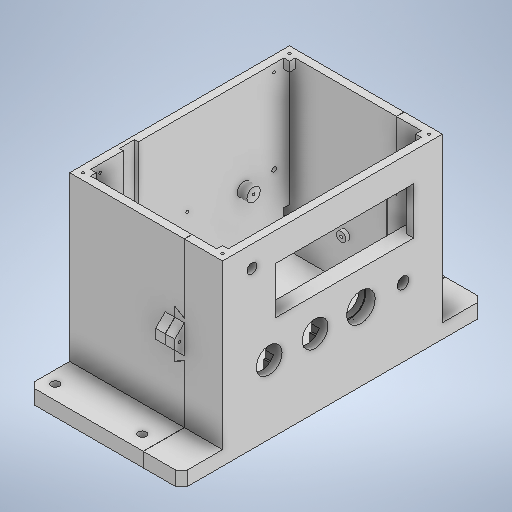
# Autodesk Inventor part: Honigschleuder_Steuerung
Saved by Autodesk Inventor 2025 (Build 290162010, 162A)
## iProperties
Created: 2025-12-04
Part Number: Honigschleuder_Steuerung
Material: Generisch
Document SubType Name: Modeling
Designer: max-h
Density: 1 g/cm^3
Appearance: Vorgabe
Author: max-h
Autodesk Inventor part; units mm, degrees
ref_plane "YZ Plane" through (0, 0, 0) normal (1, 0, 0) x (0, 1, 0)
ref_plane "XZ Plane" through (0, 0, 0) normal (0, 1, 0) x (-1, 0, 0)
ref_plane "XY Plane" through (0, 0, 0) normal (0, 0, 1) x (1, 0, 0)
sketch "Skizze1" plane through (0, 0, 0) normal (0, 1, 0) x (-1, 0, 0)
  line L0 (43.7441, 63.282) -> (-36.2559, 63.282)
  line L1 (-36.2559, 63.282) -> (-36.2559, -51.718)
  line L2 (-36.2559, -51.718) -> (43.7441, -51.718)
  line L3 (43.7441, -51.718) -> (43.7441, 63.282)
  point P0 (0, 0)
  dimension "d0" = 115
  dimension "d1" = 80
  constraints: 8 end point, 2 parallel, 1 horizontal, 1 perpendicular
  measures "d0" distance of L0.end L1.end
  measures "d1" distance of L1.end L2.end
extrude "Extrusion1" add sketch "Skizze1" along normal blind 93
shell "Wandung1" thickness 4 removed faces 1 at (9.5893, 93, -13.3847)
sketch "Skizze2" plane through (36.2559, 0, 63.282) normal (1, 0, 0) x (0, 0, -1)
  line L0 (27.85, 78) -> (100, 78)
  line L1 (100, 78) -> (100, 53.4)
  line L2 (100, 53.4) -> (27.85, 53.4)
  line L3 (27.85, 53.4) -> (27.85, 78)
  line L4 (115, 0) -> (115, 93) projected
  line L5 (0, 0) -> (115, 0) projected
  circle A0 centre (94.375, 35.9) radius 3
  circle A1 centre (72.375, 35.9) radius 7
  circle A2 centre (48.375, 35.9) radius 6.75
  circle A3 centre (24.375, 35.9) radius 6.75
  line L6 (27.85, 78) -> (17.85, 78) construction
  line L7 (17.85, 78) -> (17.85, 43) construction
  line L8 (17.85, 43) -> (27.85, 43) construction
  line L9 (27.85, 43) -> (27.85, 78) construction
  line L10 (94.375, 35.9) -> (24.375, 35.9) construction
  line L11 (0, 93) -> (115, 93) projected
  line L12 (0, 0) -> (0, 93) projected
  line L13 (17.625, 40.8928) -> (17.625, 21.6445) construction
  line L14 (97.375, 42.4272) -> (97.375, 31.7493) construction
  line L15 (94.375, 35.9) -> (97.375, 35.9) construction
  line L16 (24.375, 35.9) -> (17.625, 35.9) construction
  line L17 (57.5, 46.1925) -> (57.5, 22.2697) construction
  line L18 (0, 44.5) -> (0, 23.5685) construction
  line L19 (115, 44.5) -> (115, 22.2697) construction
  circle A4 centre (15.35, 82) radius 2.55
  point P0 (63.282, 0)
  dimension "d11" = 6
  dimension "d5" = 72.15
  dimension "d6" = 24.6
  dimension "d7" = 15
  dimension "d12" = 14
  dimension "d13" = 13.5
  dimension "d16" = 10
  dimension "d17" = 24
  dimension "d18" = 24
  dimension "d19" = 22
  dimension "d38" = 17.5
  dimension "d45" = 15
  dimension "d256" = 5.1
  dimension "d257" = 12.5
  dimension "d258" = 4
  constraints: 32 end point, 6 point on line, 5 vertical, 4 parallel, 4 perpendicular, 3 centre point, 3 horizontal, 2 horizontal alignment, 1 coincident, 7 other
  measures "d5" distance of L0.start L0.end
  measures "d6" distance of L2.end L0.start
  measures "d7" distance between parallel lines of L4 L1
  measures "d12" diameter of A1
  measures "d13" diameter of A2
  measures "d16" distance of L0.start L6.end
  measures "d17" distance of A2.centre point (24.375, 35.9)
  measures "d18" distance of A1.centre A2.centre
  measures "d19" distance of L10.start A1.centre
  measures "d38" distance from line of L2 A2.centre
  measures "d45" distance between parallel lines of L11 L0
  measures "d256" diameter of A4
  measures "d257" distance from line of L3 A4.centre
  measures "d258" distance from line of L0 A4.centre
extrude "Extrusion2" cut sketch "Skizze2" against normal blind 4 contours L0 L1 L2 L3 | A0 | A1 | A2 | A3 | A4
sketch "Skizze5" plane through (32.2559, 4, 59.282) normal (-1, 0, 0) x (0, 0, 1)
  line L0 (-107, 81) -> (-19.35, 81)
  line L1 (-107, 74) -> (-23.85, 74)
  line L2 (-23.85, 49.4) -> (-107, 49.4)
  line L3 (-107, 81) -> (-107, 74)
  line L4 (-23.85, 74) -> (-23.85, 69)
  line L5 (-23.85, 69) -> (-19.35, 69)
  line L6 (-19.35, 69) -> (-19.35, 81)
  line L7 (-23.85, 49.4) -> (-23.85, 55.4)
  line L8 (-23.85, 55.4) -> (-19.35, 55.4)
  line L9 (-19.35, 55.4) -> (-19.35, 43.4)
  line L10 (-23.85, 74) -> (-23.85, 49.4) projected
  line L11 (-107, 0) -> (-107, 89) projected
  circle A0 centre (-20.375, 31.9) radius 6.75 projected
  circle A1 centre (-44.375, 31.9) radius 6.75 projected
  line L12 (-8.375, 43.4) -> (-8.375, 10.9)
  line L13 (-50.575, 38.1) -> (-38.175, 38.1)
  line L14 (-38.175, 38.1) -> (-38.175, 25.7)
  line L15 (-50.575, 25.7) -> (-50.575, 38.1)
  line L16 (-26.575, 38.1) -> (-14.175, 38.1)
  line L17 (-14.175, 38.1) -> (-14.175, 25.7)
  line L18 (-26.575, 25.7) -> (-26.575, 38.1)
  line L19 (-20.375, 36.2236) -> (-20.375, 29.8227)
  line L20 (-44.375, 34.0681) -> (-44.375, 29.7319)
  line L21 (-22.4882, 31.9) -> (-18.3084, 31.9)
  line L22 (-47.5123, 31.9) -> (-42.4971, 31.9)
  line L23 (-49.575, 10.9) -> (-49.575, 25.7)
  line L24 (-49.575, 25.7) -> (-50.575, 25.7)
  line L25 (-38.175, 25.7) -> (-39.175, 25.7)
  line L26 (-39.175, 25.7) -> (-39.175, 10.9)
  line L27 (-39.175, 10.9) -> (-25.575, 10.9)
  line L28 (-25.575, 10.9) -> (-25.575, 25.7)
  line L29 (-25.575, 25.7) -> (-26.575, 25.7)
  line L30 (-14.175, 25.7) -> (-15.175, 25.7)
  line L31 (-15.175, 25.7) -> (-15.175, 10.9)
  line L32 (-15.175, 10.9) -> (-8.375, 10.9)
  line L33 (-8.375, 43.4) -> (-19.35, 43.4)
  line L34 (-107, 10.9) -> (-107, 49.4)
  circle A2 centre (-68.375, 31.9) radius 7 projected
  line L35 (-61.4875, 33.15) -> (-58.9875, 33.15)
  line L36 (-58.9875, 33.15) -> (-58.9875, 30.65)
  line L37 (-58.9875, 30.65) -> (-61.375, 30.65)
  circle A3 centre (-90.375, 31.9) radius 3 projected
  line L38 (-75.375, 31.9) -> (-61.375, 31.9) construction
  line L39 (-75.375, 10.9) -> (-75.375, 20.65)
  line L40 (-49.575, 10.9) -> (-61.375, 10.9)
  line L41 (-75.375, 10.9) -> (-107, 10.9)
  line L42 (-96.975, 38.4) -> (-83.775, 38.4)
  line L43 (-83.775, 38.4) -> (-83.775, 25.4)
  line L44 (-83.775, 25.4) -> (-96.975, 25.4)
  line L45 (-96.975, 25.4) -> (-96.975, 38.4)
  line L46 (-91.4544, 31.9) -> (-89.4789, 31.9)
  line L47 (-90.375, 32.9395) -> (-90.375, 31.2421)
  line L48 (-61.375, 31.9) -> (-61.375, 30.65) construction
  line L49 (-61.375, 30.65) -> (-61.375, 20.65) construction
  line L50 (-61.375, 30.65) -> (-61.4875, 30.65)
  line L51 (-61.375, 31.9) -> (-59.9359, 31.9) construction
  line L52 (-75.375, 20.65) -> (-61.375, 20.65)
  line L53 (-61.375, 20.65) -> (-61.375, 10.9)
  line L54 (-75.375, 20.65) -> (-75.375, 31.9) construction
  circle A4 centre (-72.875, 23.65) radius 0.5
  circle A5 centre (-68.375, 23.65) radius 0.5
  circle A6 centre (-63.875, 23.65) radius 0.5
  line L55 (-72.875, 23.65) -> (-63.875, 23.65) construction
  circle A7 centre (-68.375, 31.9) radius 7 construction
  line L56 (-68.375, 23.65) -> (-68.375, 31.9) construction
  point P0 (-59.282, -4)
  point P1 (-50.575, 29.2312)
  point P2 (-50.575, 34.5688)
  point P3 (-47.0438, 38.1)
  point P4 (-41.7062, 38.1)
  point P5 (-38.175, 34.5688)
  point P6 (-38.175, 29.2312)
  point P7 (-26.575, 29.2312)
  point P8 (-26.575, 34.5688)
  point P9 (-23.0438, 38.1)
  point P10 (-17.7062, 38.1)
  point P11 (-14.175, 34.5688)
  point P12 (-14.175, 29.2312)
  point P13 (-107, 49.4)
  dimension "d24" = 7
  dimension "d26" = 12
  dimension "d28" = 4.5
  dimension "d39" = 12
  dimension "d42" = 12.4
  dimension "d43" = 1
  dimension "d44" = 21
  dimension "d46" = 12
  dimension "d59" = 6
  dimension "d61" = 2.5
  dimension "d62" = 2.5
  dimension "d66" = 13.2
  dimension "d67" = 13
  dimension "d68" = 11.8
  dimension "d91" = 10
  dimension "d92" = 7
  dimension "d93" = 2.5
  dimension "d94" = 2.5
  dimension "d95" = 1
  constraints: 111 end point, 25 perpendicular, 15 horizontal, 10 point on line, 8 equal length, 7 parallel, 5 collinear, 4 point on circle, 4 vertical, 3 centre point, 3 midpoint, 3 tangent, 2 equal radius, 7 other
  measures "d24" distance between parallel lines of L0 L1
  measures "d26" distance of L5.end L0.end
  measures "d28" distance of L4.end L5.end
  measures "d39" distance from line of L12 A0.centre
  measures "d42" distance of L16.start L16.end
  measures "d43" distance of L28.end L18.start
  measures "d44" distance from line of L27 A1.centre
  measures "d46" distance of L8.end L9.end
  measures "d59" distance of L2.start L7.end
  measures "d61" distance of L36.end L50.end
  measures "d62" distance of L35.end L36.end
  measures "d66" distance of L42.start L42.end
  measures "d67" distance of L42.end L43.end
  measures "d68" distance of L23.start L40.end
  measures "d91" distance between parallel lines of L37 L52
  measures "d92" distance between parallel lines of L37 L55
  measures "d93" distance from line of L54 L55.start
  measures "d94" distance from line of L53 L55.end
  measures "d95" diameter of A4
extrude "Extrusion4" add sketch "Skizze5" along normal blind 4 contours L0 L6 L5 L4 L1 L3 | L2 L7 L8 L9 L33 L12 L32 L31 L30 L17 A0 L16 L18 L29 L28 L27 L26 L25 L14 A1 L13 L15 L24 L23 L40 L53 L52 L39 L41 L11
sketch "Skizze6" plane through (28.2559, 4, 59.282) normal (-1, 0, 0) x (0, 0, 1)
  circle A0 centre (-97.425, 77.3) radius 1
  circle A1 centre (-22.425, 77.3) radius 1
  circle A2 centre (-22.425, 46.7) radius 1
  circle A3 centre (-97.425, 46.7) radius 1
  line L0 (-22.425, 77.3) -> (-97.425, 77.3) construction
  line L1 (-97.425, 77.3) -> (-97.425, 46.7) construction
  line L2 (-97.425, 46.7) -> (-22.425, 46.7) construction
  line L3 (-22.425, 46.7) -> (-22.425, 77.3) construction
  line L4 (-107, 74) -> (-23.85, 74) construction
  line L5 (-96, 49.4) -> (-96, 74) construction
  circle A4 centre (-53.575, 17.7) radius 1
  circle A5 centre (-35.175, 17.7) radius 1
  circle A6 centre (-29.575, 17.7) radius 1
  circle A7 centre (-11.175, 17.7) radius 1
  line L6 (-53.575, 17.7) -> (-11.175, 17.7) construction
  line L7 (-14.175, 38.1) -> (-14.175, 25.7) construction
  line L8 (-26.575, 25.7) -> (-26.575, 38.1) construction
  line L9 (-38.175, 38.1) -> (-38.175, 25.7) construction
  line L10 (-50.575, 25.7) -> (-50.575, 38.1) construction
  line L11 (-39.175, 10.9) -> (-25.575, 10.9) construction
  line L12 (-38.175, 25.7) -> (-39.175, 25.7) construction
  line L13 (-23.85, 49.4) -> (-107, 49.4) projected
  point P0 (-59.282, -4)
  point P1 (-38.675, 25.7)
  point P2 (-14.175, 34.5688)
  point P3 (-14.175, 29.2312)
  point P4 (-26.575, 29.2312)
  point P5 (-26.575, 34.5688)
  point P6 (-38.175, 34.5688)
  point P7 (-38.175, 29.2312)
  point P8 (-50.575, 29.2312)
  point P9 (-50.575, 34.5688)
  dimension "d31" = 75
  dimension "d32" = 30.6
  dimension "d33" = 2
  dimension "d35" = 1.425
  dimension "d48" = 3
  dimension "d49" = 3
  dimension "d50" = 3
  dimension "d51" = 3
  dimension "d52" = 8
  dimension "d77" = 2.7
  constraints: 10 end point, 8 centre point, 7 equal radius, 3 parallel, 2 coincident, 2 point on line, 1 horizontal, 1 midpoint, 1 perpendicular
  measures "d31" distance of L0.start A0.centre
  measures "d32" distance of L2.end L0.start
  measures "d33" diameter of A1
  measures "d35" distance between parallel lines of L5 L1
  measures "d48" distance from line of L6.end L7
  measures "d49" distance from line of L8 A6.centre
  measures "d50" distance from line of L9 A5.centre
  measures "d51" distance from line of L10 L6.start
  measures "d52" distance from line of point (-38.675, 25.7) L6
  measures "d77" distance between parallel lines of L13 L2
extrude "Extrusion5" cut sketch "Skizze6" against normal blind 3
sketch "Skizze8" plane through (32.2559, 4, 59.282) normal (-1, 0, 0) x (0, 0, 1)
  line L0 (-49.575, 25.7) -> (-49.575, 10.9) projected
  line L1 (0, 0) -> (-107, 0) projected
  line L2 (-49.575, 22.7) -> (-39.175, 22.7)
  line L3 (-39.175, 22.7) -> (-39.175, 0)
  line L4 (-39.175, 0) -> (-49.575, 0)
  line L5 (-49.575, 0) -> (-49.575, 22.7)
  line L6 (-25.575, 22.7) -> (-15.175, 22.7)
  line L7 (-15.175, 22.7) -> (-15.175, 0)
  line L8 (-15.175, 0) -> (-25.575, 0)
  line L9 (-25.575, 0) -> (-25.575, 22.7)
  line L10 (-39.175, 10.9) -> (-39.175, 25.7) projected
  line L11 (-25.575, 25.7) -> (-25.575, 10.9) projected
  line L12 (-15.175, 10.9) -> (-15.175, 25.7) projected
  point P0 (-59.282, -4)
  point P1 (-46.65, 8.9)
  point P2 (-25.575, 0)
  point P3 (-49.575, 0)
  dimension "d63" = 3
  constraints: 16 end point, 5 point on line, 4 parallel, 2 horizontal, 2 perpendicular, 1 collinear, 2 other
  measures "d63" distance from line of point (-49.575, 25.7) L2
extrude "Extrusion7" cut sketch "Skizze8" against normal blind 2
sketch "Skizze12" plane through (-39.7441, 4, -47.718) normal (1, 0, 0) x (0, 0, -1)
  circle A0 centre (-23.75, 40) radius 3.5
  circle A1 centre (-97.5, 74.5) radius 3.5
  line L0 (0, 0) -> (-107, 0) projected
  line L1 (0, 0) -> (0, 89) projected
  line L2 (-107, 0) -> (-107, 89) projected
  line L3 (-107, 89) -> (0, 89) projected
  circle A2 centre (-97.5, 21.5) radius 3.5
  line L4 (-97.5, 74.5) -> (-97.5, 21.5) construction
  point P0 (-47.718, -4)
  dimension "d99" = 9.5
  dimension "d100" = 14.5
  dimension "d101" = 7
  dimension "d165" = 53
  dimension "d196" = 49
  dimension "d235" = 73.75
  constraints: 3 centre point, 2 end point, 2 equal radius, 1 parallel
  measures "d99" distance from line of L2 L4.start
  measures "d100" distance from line of L3 L4.start
  measures "d101" diameter of A1
  measures "d165" distance of L4.start L4.end
  measures "d196" distance from line of L3 A0.centre
  measures "d235" horizontal distance of A0.centre L4.start
extrude "Extrusion11" add sketch "Skizze12" along normal blind 5 contours A0 | A1 | A2
sketch "Skizze13" plane through (-34.7441, 78.5, 49.782) normal (1, 0, 0) x (0, 0, -1)
  circle A0 centre (0, 0) radius 0.7
  circle A1 centre (73.75, -34.5) radius 3.5 projected
  circle A2 centre (73.75, -34.5) radius 0.7
  circle A3 centre (0, -53) radius 3.5 projected
  circle A4 centre (0, -53) radius 0.7
  circle A5 centre (0, 0) radius 3.5 projected
  point P0 (49.782, -78.5)
  dimension "d104" = 1.4
  constraints: 3 centre point, 3 coincident, 2 equal radius
  measures "d104" diameter of A0
extrude "Extrusion12" cut sketch "Skizze13" against normal blind 5 contours A0 | A2 | A4
sketch "Skizze20" plane through (0, 93, 0) normal (0, 1, 0) x (1, 0, 0)
  line L0 (36.2559, 51.718) -> (-43.7441, 51.718) projected
  line L1 (-43.7441, 51.718) -> (-36.7441, 51.718)
  line L2 (-36.7441, 51.718) -> (-36.7441, 44.718)
  line L3 (-36.7441, 44.718) -> (-43.7441, 44.718)
  line L4 (-43.7441, 44.718) -> (-43.7441, 51.718)
  line L5 (36.2559, 51.718) -> (29.2559, 51.718)
  line L6 (29.2559, 51.718) -> (29.2559, 44.718)
  line L7 (29.2559, 44.718) -> (36.2559, 44.718)
  line L8 (36.2559, 44.718) -> (36.2559, 51.718)
  line L9 (36.2559, -63.282) -> (29.2559, -63.282)
  line L10 (29.2559, -63.282) -> (29.2559, -56.282)
  line L11 (29.2559, -56.282) -> (36.2559, -56.282)
  line L12 (36.2559, -56.282) -> (36.2559, -63.282)
  line L13 (-43.7441, 51.718) -> (-43.7441, -63.282) projected
  line L14 (-43.7441, -63.282) -> (-36.7441, -63.282)
  line L15 (-36.7441, -63.282) -> (-36.7441, -56.282)
  line L16 (-36.7441, -56.282) -> (-43.7441, -56.282)
  line L17 (-43.7441, -56.282) -> (-43.7441, -63.282)
  point P0 (0, 0)
  point P1 (-43.7441, 6.718)
  point P2 (-43.7441, -56.282)
  point P3 (29.2559, 51.718)
  dimension "d136" = 7
  constraints: 32 end point, 8 parallel, 7 equal length, 4 horizontal, 4 perpendicular, 1 point on line
  measures "d136" distance of L2.end L3.end
extrude "Extrusion19" add sketch "Skizze20" against normal blind 8
sketch "Skizze21" plane through (0, 93, 0) normal (0, 1, 0) x (1, 0, 0)
  circle A0 centre (-40.2441, -59.782) radius 0.7
  circle A1 centre (-40.2441, 48.218) radius 0.7
  circle A2 centre (32.7559, 48.218) radius 0.7
  circle A3 centre (32.7559, -59.782) radius 0.7
  line L0 (-43.7441, -63.282) -> (36.2559, -63.282) projected
  line L1 (36.2559, -63.282) -> (36.2559, 51.718) projected
  line L2 (36.2559, 51.718) -> (-43.7441, 51.718) projected
  line L3 (-43.7441, 51.718) -> (-43.7441, -63.282) projected
  line L4 (-36.7441, -59.282) -> (-36.7441, -56.282) projected
  line L5 (-36.7441, -56.282) -> (-39.7441, -56.282) projected
  line L6 (-39.7441, -56.282) -> (-39.7441, 44.718) projected
  line L7 (-39.7441, 44.718) -> (-36.7441, 44.718) projected
  line L8 (-36.7441, 44.718) -> (-36.7441, 47.718) projected
  line L9 (-36.7441, 47.718) -> (29.2559, 47.718) projected
  line L10 (29.2559, 47.718) -> (29.2559, 44.718) projected
  line L11 (29.2559, 44.718) -> (32.2559, 44.718) projected
  line L12 (32.2559, 44.718) -> (32.2559, -56.282) projected
  line L13 (32.2559, -56.282) -> (29.2559, -56.282) projected
  line L14 (29.2559, -56.282) -> (29.2559, -59.282) projected
  line L15 (29.2559, -59.282) -> (-36.7441, -59.282) projected
  line L16 (-40.2441, -59.782) -> (32.7559, -59.782) construction
  line L17 (32.7559, -59.782) -> (32.7559, 48.218) construction
  line L18 (32.7559, 48.218) -> (-40.2441, 48.218) construction
  line L19 (-40.2441, 48.218) -> (-40.2441, -59.782) construction
  point P0 (0, 0)
  dimension "d139" = 3.5
  dimension "d140" = 1.4
  constraints: 8 end point, 4 centre point, 4 coincident, 3 equal radius, 3 other
  measures "d139" distance between parallel lines of L3 L19
  measures "d140" diameter of A0
extrude "Extrusion20" cut sketch "Skizze21" against normal blind 5 contours A0 | A1 | A2 | A3
chamfer "Fasen1" distance 3 angle 45 6 edges at (-36.7441, 85, -46.218) (-38.2441, 85, -44.718) (30.7559, 85, 56.282) (29.2559, 85, 57.782) (-38.2441, 85, 56.282) (-36.7441, 85, 57.782)
sketch "Skizze22" plane through (-43.7441, 0, 63.282) normal (0, 0, 1) x (1, 0, 0)
  line L0 (50, 50) -> (60, 50)
  line L1 (60, 50) -> (60, 45)
  line L2 (60, 45) -> (50, 45)
  line L3 (50, 45) -> (50, 50)
  line L4 (80, 0) -> (80, 93) projected
  line L5 (0, 93) -> (80, 93) projected
  point P0 (43.7441, 0)
  dimension "d146" = 10
  dimension "d147" = 5
  dimension "d148" = 20
  dimension "d149" = 43
  constraints: 8 end point, 2 parallel, 1 horizontal, 1 perpendicular
  measures "d146" distance of L0.start L0.end
  measures "d147" distance of L0.end L1.end
  measures "d148" distance between parallel lines of L4 L1
  measures "d149" distance between parallel lines of L5 L0
extrude "Extrusion21" add sketch "Skizze22" along normal blind 5
sketch "Skizze23" plane through (36.2559, 93, -51.718) normal (0, 0, -1) x (-1, 0, 0)
  line L0 (20, -43) -> (30, -43) projected
  line L1 (20, -48) -> (20, -43) projected
  line L2 (30, -48) -> (20, -48) projected
  line L3 (30, -43) -> (30, -48) projected
  point P0 (36.2559, -93)
extrude "Extrusion22" add sketch "Skizze23" along normal blind 5
sketch "Skizze24" plane through (16.2559, 45, -51.718) normal (1, 0, 0) x (0, 0, -1)
  circle A0 centre (2.5, 2.5) radius 0.7
  line L0 (5, 5) -> (5, 0) projected
  line L1 (0, 5) -> (5, 5) projected
  circle A1 centre (-117.5, 2.5) radius 0.7
  line L2 (-115, 5) -> (-120, 5) projected
  line L3 (-120, 0) -> (-120, 5) projected
  point P0 (-51.718, -45)
  point P1 (2.5, 5)
  point P2 (-120, 2.5)
  dimension "d154" = 2.5
  dimension "d155" = 2.5
  dimension "d156" = 1.4
  dimension "d157" = 2.5
  dimension "d158" = 2.5
  dimension "d159" = 1.4
  constraints: 2 centre point, 2 midpoint
  measures "d154" distance from line of L0 A0.centre
  measures "d155" distance of point (2.5, 5) A0.centre
  measures "d156" diameter of A0
  measures "d157" distance from line of L2 A1.centre
  measures "d158" distance of point (-120, 2.5) A1.centre
  measures "d159" diameter of A1
extrude "Extrusion23" cut sketch "Skizze24" against normal blind 10
chamfer "Fasen2" distance 5 angle 45 4 edges at (11.2559, 50, 63.282) (11.2559, 45, 63.282) (11.2559, 50, -51.718) (11.2559, 45, -51.718)
sketch "Skizze25" plane through (36.2559, 0, 63.282) normal (1, 0, 0) x (0, 0, -1)
  circle A0 centre (72.375, 35.9) radius 7 projected
  circle A1 centre (72.375, 35.9) radius 7.5
  point P0 (63.282, 0)
  dimension "d166" = 0.5
  constraints: 1 centre point, 1 coincident
  measures "d166" radial gap between concentric circles of A0 A1
extrude "Extrusion24" cut sketch "Skizze25" against normal blind 5
sketch "Skizze27" plane through (28.2559, 4, 59.282) normal (-1, 0, 0) x (0, 0, 1)
  line L0 (-48.125, 40.1) -> (-40.625, 40.1)
  line L1 (-40.625, 40.1) -> (-40.625, 38.1)
  line L2 (-40.625, 38.1) -> (-48.125, 38.1)
  line L3 (-48.125, 38.1) -> (-48.125, 40.1)
  line L4 (-24.125, 40.1) -> (-16.625, 40.1)
  line L5 (-16.625, 40.1) -> (-16.625, 38.1)
  line L6 (-16.625, 38.1) -> (-24.125, 38.1)
  line L7 (-24.125, 38.1) -> (-24.125, 40.1)
  line L8 (-44.375, 46.4006) -> (-44.375, 32.378)
  line L9 (-20.375, 42.4036) -> (-20.375, 30.1391)
  arc A0 (-38.175, 29.2312) -> (-38.175, 34.5688) centre (-44.375, 31.9) ccw projected
  arc A1 (-14.175, 29.2312) -> (-14.175, 34.5688) centre (-20.375, 31.9) ccw projected
  line L10 (-50.575, 38.1) -> (-47.0438, 38.1) projected
  point P0 (-59.282, -4)
  dimension "d169" = 7.5
  dimension "d170" = 2
  constraints: 20 end point, 4 parallel, 3 point on line, 2 equal length, 2 horizontal, 2 perpendicular, 2 vertical, 1 collinear, 2 other
  measures "d169" distance of L0.start L0.end
  measures "d170" distance of L0.end L1.end
extrude "Extrusion25" cut sketch "Skizze27" against normal blind 2
sketch "Skizze28" plane through (-39.7441, 4, 59.282) normal (1, 0, 0) x (0, 0, -1)
  line L0 (107, 0) -> (0, 0) construction
  line L1 (0, 0) -> (0, 89) construction
  line L2 (0, 89) -> (107, 89) construction
  line L3 (107, 89) -> (107, 0) construction
  line L4 (0, 0) -> (0, 81) projected
  line L5 (107, 0) -> (0, 0) projected
  line L6 (107, 0) -> (107, 81) projected
  line L7 (104, 84) -> (107, 81) projected
  line L8 (104, 84) -> (104, 89) projected
  line L9 (3, 89) -> (104, 89) projected
  line L10 (3, 89) -> (3, 84) projected
  line L11 (0, 81) -> (3, 84) projected
  circle A0 centre (9.5, 74.5) radius 3.5 projected
  circle A1 centre (83.25, 40) radius 3.5 projected
  circle A2 centre (9.5, 21.5) radius 3.5 projected
  line L12 (103, 85) -> (4, 85) construction
  line L13 (4, 85) -> (4, 4) construction
  line L14 (4, 4) -> (103, 4) construction
  line L15 (103, 4) -> (103, 85) construction
  circle A3 centre (4, 85) radius 0.7 construction
  circle A4 centre (103, 85) radius 0.7 construction
  circle A5 centre (103, 4) radius 0.7
  circle A6 centre (4, 4) radius 0.7
  line L16 (107, 89) -> (107, 49.8) construction
  line L17 (107, 0) -> (107, 81) projected
  line L18 (3, 89) -> (104, 89) projected
  line L19 (0, 0) -> (0, 81) projected
  circle A7 centre (8, 85) radius 0.7
  circle A8 centre (99, 85) radius 0.7
  line L20 (4, 85) -> (103, 4) construction
  line L21 (4, 4) -> (103, 85) construction
  circle A9 centre (53.5, 44.5) radius 0.7
  point P0 (59.282, -4)
  dimension "d175" = 4
  dimension "d176" = 1.4
  dimension "d218" = 4
  dimension "d219" = 4
  constraints: 22 end point, 7 centre point, 6 equal radius, 5 point on line, 4 coincident, 4 parallel, 2 perpendicular, 1 horizontal, 1 midpoint, 3 other
  measures "d175" distance between parallel lines of L2 L12
  measures "d176" diameter of A3
  measures "d218" distance of L12.end A7.centre
  measures "d219" distance of L12.start A8.centre
extrude "Extrusion26" cut sketch "Skizze28" against normal blind 4 contours A5 | A6 | A7 | A8 | A9
sketch "Skizze29" plane through (-43.7441, 0, 63.282) normal (0, 0, 1) x (1, 0, 0)
  line L0 (0, 0) -> (0, 93) projected
  line L1 (0, 0) -> (80, 0)
  line L2 (80, 0) -> (80, 7.5)
  line L3 (80, 7.5) -> (0, 7.5)
  line L4 (0, 7.5) -> (0, 0)
  line L5 (80, 0) -> (80, 93) projected
  line L6 (80, 0) -> (45, 0)
  line L7 (80, 7.5) -> (80, 0)
  point P0 (43.7441, 0)
  point P1 (0, 7.5)
  dimension "d181" = 7.5
  constraints: 12 end point, 2 horizontal, 2 parallel, 1 perpendicular, 1 point on line
  measures "d181" distance of L1.end L2.end
extrude "Extrusion27" add sketch "Skizze29" along normal blind 21.5
sketch "Skizze30" plane through (36.2559, 0, -51.718) normal (0, 0, -1) x (-1, 0, 0)
  line L0 (0, 7.5) -> (80, 7.5) projected
  line L1 (80, 7.5) -> (80, 0) projected
  line L2 (80, 0) -> (0, 0) projected
  line L3 (0, 0) -> (0, 7.5) projected
  point P0 (36.2559, 0)
extrude "Extrusion28" add sketch "Skizze30" along normal blind 21.5
chamfer "Fasen3" distance 3 angle 45 4 edges at (-43.7441, 3.75, 84.782) (36.2559, 3.75, 84.782) (36.2559, 3.75, -73.218) (-43.7441, 3.75, -73.218)
sketch "Skizze32" plane through (-39.7441, 4, 59.282) normal (1, 0, 0) x (0, 0, -1)
  line L0 (107, 0) -> (0, 0) projected
  line L1 (28, 0) -> (20, 0)
  line L2 (20, 0) -> (20, 4)
  line L3 (20, 4) -> (28, 4)
  line L4 (28, 4) -> (28, 0)
  line L5 (0, 0) -> (0, 81) projected
  point P0 (59.282, -4)
  point P1 (20, 0)
  dimension "d197" = 8
  dimension "d198" = 4
  dimension "d199" = 20
  constraints: 8 end point, 2 parallel, 1 horizontal, 1 perpendicular, 1 point on line
  measures "d197" distance of L2.end L3.end
  measures "d198" distance of L3.end L1.start
  measures "d199" distance between parallel lines of L5 L2
extrude "Extrusion30" cut sketch "Skizze32" against normal blind 5
sketch "Skizze33" plane through (-39.7441, 93, 56.282) normal (1, 0, 0) x (0, 0, -1)
  line L0 (17, -85) -> (25, -85) projected
  line L1 (0, 0) -> (101, 0) projected
  line L2 (25, -85) -> (17, -85)
  line L3 (17, -85) -> (17, 0)
  line L4 (17, 0) -> (25, 0)
  line L5 (25, 0) -> (25, -85)
  point P0 (56.282, -93)
  point P1 (25, 0)
  constraints: 8 end point, 2 parallel, 1 horizontal, 1 perpendicular, 1 point on line
extrude "Extrusion31" cut sketch "Skizze33" against normal blind 2
sketch "Skizze34" plane through (-43.7441, 7.5, 63.282) normal (0, 1, 0) x (1, 0, 0)
  circle A0 centre (6.5, -14) radius 2.1
  circle A1 centre (52, -14) radius 2.1
  circle A2 centre (6.5, 129) radius 2.1
  circle A3 centre (52, 129) radius 2.1
  line L0 (6.5, -14) -> (52, -14) construction
  line L1 (52, -14) -> (52, 129) construction
  line L2 (52, 129) -> (6.5, 129) construction
  line L3 (6.5, 129) -> (6.5, -14) construction
  line L4 (77, -21.5) -> (3, -21.5) construction
  line L5 (3, 136.5) -> (77, 136.5) construction
  line L6 (80, 0) -> (80, -18.5) construction
  point P0 (43.7441, 63.282)
  point P1 (80, -9.25)
  dimension "d204" = 4.2
  dimension "d205" = 7.5
  dimension "d206" = 7.5
  dimension "d207" = 28
  dimension "d208" = 45.5
  constraints: 8 end point, 4 centre point, 3 equal radius, 2 coincident, 2 parallel, 1 horizontal, 1 midpoint, 1 perpendicular
  measures "d204" diameter of A0
  measures "d205" distance between parallel lines of L4 L0
  measures "d206" distance between parallel lines of L5 L2
  measures "d207" distance from line of point (80, -9.25) L1
  measures "d208" distance of L0.start L0.end
extrude "Extrusion32" cut sketch "Skizze34" against normal through all
sketch "Skizze35" plane through (-43.7441, 93, -51.718) normal (-1, 0, 0) x (0, 0, 1)
  line L0 (95.825, -89) -> (85.425, -89) projected
  line L1 (133.5, -93) -> (-18.5, -93) projected
  line L2 (91, -89) -> (83, -89)
  line L3 (83, -89) -> (83, -93)
  line L4 (83, -93) -> (91, -93)
  line L5 (91, -93) -> (91, -89)
  point P0 (51.718, -93)
  constraints: 8 end point, 2 parallel, 1 coincident, 1 horizontal, 1 perpendicular, 1 point on line
extrude "Extrusion33" cut sketch "Skizze35" against normal blind 4
chamfer "Fasen4" distance 2 angle 45 1 edges at (-39.7441, 4, 35.282)
sketch "Skizze36" plane through (-43.7441, 0, 84.782) normal (0, 0, 1) x (1, 0, 0)
  line L0 (60, 93) -> (60, 57.1132) construction
  line L1 (60, 57.1132) -> (55, 60) construction
  line L2 (55, 60) -> (55, 35) construction
  line L3 (55, 35) -> (60, 37.8868) construction
  line L4 (60, 37.8868) -> (60, 0) construction
  line L5 (0, 93) -> (80, 93) projected
  line L6 (3, 0) -> (77, 0) projected
  line L7 (50, 50) -> (50, 45) projected
  line L8 (60, 45) -> (60, 50) projected
  line L9 (60, 50) -> (50, 50) projected
  line L10 (59.94, 0) -> (59.94, 37.7828)
  line L11 (59.94, 37.7828) -> (54.94, 34.8961)
  line L12 (54.94, 34.8961) -> (54.94, 60.1039)
  line L13 (54.94, 60.1039) -> (59.94, 57.2172)
  line L14 (59.94, 57.2172) -> (59.94, 93)
  line L15 (60.06, 0) -> (60.06, 37.9907)
  line L16 (60.06, 37.9907) -> (55.06, 35.1039)
  line L17 (55.06, 35.1039) -> (55.06, 59.8961)
  line L18 (55.06, 59.8961) -> (60.06, 57.0093)
  line L19 (60.06, 57.0093) -> (60.06, 93)
  point P0 (43.7441, 0)
  point P1 (59.94, 0)
  point P2 (60.06, 0)
  dimension "d220" = 60
  dimension "d221" = 60
  dimension "d222" = 5
  dimension "d223" = 25
  dimension "d224" = 5
  dimension "d225" = 10
  dimension "d226" = 0.06
  dimension "d227" = 0.06
  constraints: 30 end point, 4 point on line, 3 parallel, 1 vertical, 8 other
  measures "d220" angle of L0 L1
  measures "d221" angle of L4 L3
  measures "d222" distance between parallel lines of L0 L2
  measures "d223" distance of L1.end L2.end
  measures "d224" distance between parallel lines of L7 L2
  measures "d225" distance from line of L9 L1.end
  measures "d226" distance between parallel lines of L2 L12
  measures "d227" distance between parallel lines of L2 L17
extrude "Extrusion34" cut sketch "Skizze36" against normal through all
sketch "Skizze37" plane through (-43.7441, 93, -51.718) normal (-1, 0, 0) x (0, 0, 1)
  circle A0 centre (12, -48) radius 1.2
  line L0 (83, -93) -> (-18.5, -93) projected
  line L1 (0, -85.5) -> (0, 0) projected
  point P0 (51.718, -93)
  dimension "d230" = 45
  dimension "d231" = 12
  dimension "d232" = 2.4
  constraints: 1 centre point
  measures "d230" distance from line of L0 A0.centre
  measures "d231" distance from line of L1 A0.centre
  measures "d232" diameter of A0
extrude "Extrusion35" cut sketch "Skizze37" against normal blind 10
sketch "Skizze38" plane through (-39.7441, 4, -47.718) normal (1, 0, 0) x (0, 0, -1)
  line L0 (-3, 21) -> (0, 21)
  line L1 (0, 21) -> (0, 15)
  line L2 (0, 15) -> (-3, 15)
  line L3 (-3, 15) -> (-3, 21)
  line L4 (0, 0) -> (-79, 0) projected
  line L5 (0, 0) -> (0, 81) projected
  point P0 (-47.718, -4)
  dimension "d236" = 15
  dimension "d237" = 3
  dimension "d238" = 6
  constraints: 8 end point, 2 parallel, 1 horizontal, 1 perpendicular, 1 point on line
  measures "d236" distance between parallel lines of L4 L2
  measures "d237" distance of L1.end L2.end
  measures "d238" distance of L2.end L0.start
extrude "Extrusion36" cut sketch "Skizze38" against normal blind 21.5
sketch "Skizze39" plane through (-36.7441, 88, -47.718) normal (0, 0, 1) x (1, 0, 0)
  line L0 (45.56, -25) -> (24.06, -25) construction
  line L1 (24.06, -25) -> (24.06, -68.5) construction
  line L2 (24.06, -68.5) -> (45.56, -68.5) construction
  line L3 (45.56, -68.5) -> (45.56, -25) construction
  line L4 (53.06, 5) -> (53.06, -30.9907) projected
  line L5 (0, 5) -> (52.94, 5) projected
  circle A0 centre (43.56, -31.5) radius 2.5
  circle A1 centre (26.06, -62) radius 2.5
  point P0 (36.7441, -88)
  dimension "d241" = 7.5
  dimension "d242" = 43.5
  dimension "d243" = 21.5
  dimension "d244" = 30
  dimension "d245" = 6.5
  dimension "d247" = 2
  dimension "d248" = 2
  dimension "d249" = 6.5
  dimension "d250" = 5
  constraints: 8 end point, 2 centre point, 2 parallel, 1 equal radius, 1 horizontal, 1 perpendicular
  measures "d241" distance between parallel lines of L4 L3
  measures "d242" distance of L0.end L1.end
  measures "d243" distance of L0.start L0.end
  measures "d244" distance between parallel lines of L5 L0
  measures "d245" distance from line of L0 A0.centre
  measures "d247" distance from line of L3 A0.centre
  measures "d248" distance from line of L1 A1.centre
  measures "d249" distance from line of L2 A1.centre
  measures "d250" diameter of A0
extrude "Extrusion37" add sketch "Skizze39" along normal blind 2
sketch "Skizze41" plane through (6.8159, 56.5, -45.718) normal (0, 0, 1) x (1, 0, 0)
  circle A0 centre (0, 0) radius 2.5 projected
  circle A1 centre (0, 0) radius 0.7
  circle A2 centre (-17.5, -30.5) radius 2.5 projected
  circle A3 centre (-17.5, -30.5) radius 0.7
  point P0 (-6.8159, -56.5)
  dimension "d253" = 1.4
  constraints: 2 centre point, 2 coincident, 1 equal radius
  measures "d253" diameter of A1
extrude "Extrusion38" cut sketch "Skizze41" against normal blind 4 contours A1 | A3
